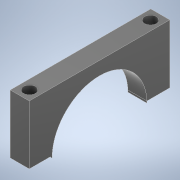
# Autodesk Inventor part: TubeClamp
Saved by Autodesk Inventor 2022 (Build 260153000, 153)
## iProperties
Created: 2022-02-05
Part Number: TubeClamp
Material: Generic
Document SubType Name: Modeling
Designer: ultra
Density: 1 g/cm^3
Appearance: Smooth - Black
Author: ultra
Autodesk Inventor part; units mm, degrees
ref_plane "YZ Plane" through (0, 0, 0) normal (1, 0, 0) x (0, 1, 0)
ref_plane "XZ Plane" through (0, 0, 0) normal (0, 1, 0) x (-1, 0, 0)
ref_plane "XY Plane" through (0, 0, 0) normal (0, 0, 1) x (1, 0, 0)
sketch "Sketch1" plane through (0, 0, 0) normal (1, 0, 0) x (0, 1, 0)
  circle A0 centre (0, 0) radius 12.5
  line L0 (0, 12.5) -> (0, -12.5)
  line L1 (0, -12.5) -> (12.5, -12.5)
  line L2 (12.5, -12.5) -> (12.5, 12.5)
  line L3 (12.5, 12.5) -> (0, 12.5)
  line L4 (12.5, 12.5) -> (16, 12.5)
  line L5 (16, 12.5) -> (16, -12.5)
  line L6 (16, -12.5) -> (12.5, -12.5)
  line L7 (12.5, -12.5) -> (12.5, 12.5)
  line L8 (16, 12.5) -> (12.5, 12.5)
  line L9 (12.5, 12.5) -> (12.5, 18.5)
  line L10 (12.5, 18.5) -> (16, 18.5)
  line L11 (16, 18.5) -> (16, 12.5)
  line L12 (16, -12.5) -> (12.5, -12.5)
  line L13 (12.5, -12.5) -> (12.5, -18.5)
  line L14 (12.5, -18.5) -> (16, -18.5)
  line L15 (16, -18.5) -> (16, -12.5)
  line L16 (12.5, 18.5) -> (12.5, 12.5)
  line L17 (12.5, -18.5) -> (12.5, -12.5)
  line L18 (16, 18.5) -> (0.5, 18.5)
  line L19 (0.5, 18.5) -> (0.5, 12.5)
  line L20 (0.5, 12.5) -> (16, 12.5)
  line L21 (16, 12.5) -> (16, 18.5)
  line L22 (16, -12.5) -> (0.5, -12.5)
  line L23 (0.5, -12.5) -> (0.5, -18.5)
  line L24 (0.5, -18.5) -> (16, -18.5)
  line L25 (16, -18.5) -> (16, -12.5)
  point P0 (12.5, 0)
  dimension "d0" = 25
  dimension "d1" = 3.5
  dimension "d2" = 25
  dimension "d3" = 6
  dimension "d4" = 6
  dimension "d15" = 15.5
  dimension "d16" = 15.5
  constraints: 52 end point, 12 parallel, 6 perpendicular, 5 horizontal, 2 point on circle, 1 centre point, 1 coincident, 1 vertical
  measures "d0" diameter of A0
  measures "d1" distance of L5.end L6.end
  measures "d2" distance of L4.end L5.end
  measures "d3" distance of L8.end L9.end
  measures "d4" distance of L13.end L12.end
  measures "d15" distance of L20.end L19.end
  measures "d16" distance of L24.end L23.end
extrude "Extrusion3" add sketch "Sketch1" along normal blind 5 contours L2 L1 A0 | L2 L4 L5 L6 | A0 L3 L2 | L13 L24 L23 L1 | L6 L15 L14 L13 | L9 L10 L11 L4 | L3 L19 L18 L9
sketch "Sketch4" plane through (0, 16, 18.5) normal (0, 1, 0) x (1, 0, 0)
  line L0 (0, 37) -> (5, 37)
  line L1 (0, 0) -> (5, 0)
  circle A0 centre (2.5, 2.5615) radius 1.5875
  circle A1 centre (2.5, 34.4385) radius 1.5875
  line L2 (0, 37) -> (0, 0) projected
  line L3 (5, 37) -> (5, 0) projected
  line L4 (0, 18.5) -> (5, 18.5)
  dimension "d23" = 3.175
  dimension "d24" = 3.175
  dimension "d27" = 2.5
  dimension "d28" = 15.9385
  dimension "d29" = 15.9385
  constraints: 6 end point, 2 centre point, 1 midpoint
  measures "d23" diameter of A0
  measures "d24" diameter of A1
  measures "d27" distance from line of L2 A0.centre
  measures "d28" distance from line of L4 A0.centre
  measures "d29" distance from line of L4 A1.centre
extrude "Extrusion5" cut sketch "Sketch4" against normal blind 20 contours A0 | A1
body "Solid2"
